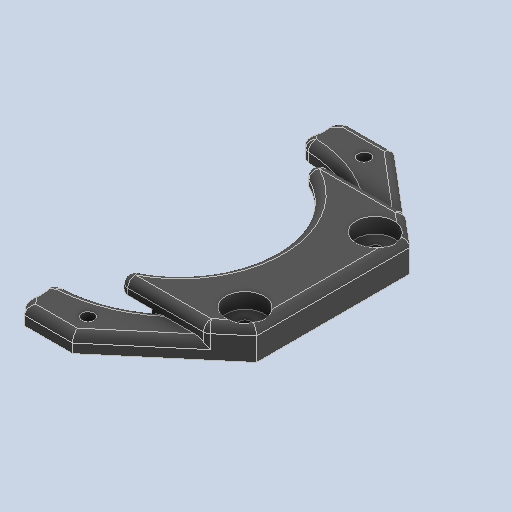
# Autodesk Inventor part: joit_cover_arm_upper
Saved by Autodesk Inventor 2026.1 (Build 301233020, 233B)
## iProperties
Created: 2024-02-14
Part Number: joit_cover_arm_upper
Material: 一般
Document SubType Name: Modeling
Designer: hibik
Density: 1 g/cm^3
Appearance: 既定
Author: hibik
Autodesk Inventor part; units mm, degrees
ref_plane "YZ Plane" through (0, 0, 0) normal (1, 0, 0) x (0, 1, 0)
ref_plane "XZ Plane" through (0, 0, 0) normal (0, 1, 0) x (-1, 0, 0)
ref_plane "XY Plane" through (0, 0, 0) normal (0, 0, 1) x (1, 0, 0)
sketch "スケッチ1" plane through (0, 0, 0) normal (0, 1, 0) x (-1, 0, 0)
  line L0 (24, 0) -> (0, 0)
  line L1 (0, 0) -> (0, -26)
  line L2 (0, -26) -> (24, -26)
  line L3 (24, -26) -> (24, 0)
  circle A0 centre (24, -13) radius 13 construction
  circle A1 centre (24, -13) radius 12.5
  circle A2 centre (24, -13) radius 16
  point P0 (24, -25.5)
  point P1 (24, -0.5)
  point P2 (14.672621, 0)
  point P3 (14.672621, -26)
  dimension "d0" = 26
  dimension "d1" = 24
  dimension "d2" = 25
  dimension "d3" = 32
  constraints: 8 end point, 3 centre point, 3 coincident, 2 parallel, 1 horizontal, 1 midpoint, 1 perpendicular, 1 tangent
  measures "d0" distance of L2.end L0.start
  measures "d1" distance of L1.end L2.end
  measures "d2" diameter of A1
  measures "d3" diameter of A2
extrude "押し出し1" add sketch "スケッチ1" along normal blind 4 contours L3 A1 L2 A2 L0 | A2 L2 L1 L0 picked at (14.087861, -23.933914)
extrude "押し出し2" cut sketch "スケッチ1" along normal blind 2.2 contours L3 A1 L2 A2 L0 picked at (14.087861, -23.933914)
fillet "フィレット1" radius 1 4 edges at (-24, 3.1, -0.5) (-24, 3.1, 0) (-24, 3.1, -26) (-24, 3.1, -25.5)
sketch "スケッチ8" plane through (0, 0, 0) normal (0, -1, 0) x (1, 0, 0)
  line L0 (-4, -3) -> (-4, -5.236068)
  line L1 (-5.661079, -1.594472) -> (-4, -3)
  line L2 (-4, -20.763932) -> (-4, -23)
  line L3 (-4, -23) -> (-5.661079, -24.405528)
  line L4 (-15.355616, -32.608598) -> (-17, -34)
  line L5 (-17, 8) -> (-15.355616, 6.608598)
  line L6 (-17, -34) -> (-45, -34)
  line L7 (-45, 8) -> (-17, 8)
  line L8 (-5.661079, -1.594472) -> (-15.355616, 6.608598)
  line L9 (-4, -5.236068) -> (-4, -20.763932)
  line L10 (-5.661079, -24.405528) -> (-15.355616, -32.608598)
  arc A0 (-18.273464, -24.111111) -> (-18.273464, -1.888889) centre (-24, -13) ccw
  circle A1 centre (-24, -13) radius 12.5
  line L11 (-23.274102, -34) -> (-25.857871, -30.946455)
  line L12 (-25.857871, -30.946455) -> (-15.925722, -22.542329)
  line L13 (-23.274102, 8) -> (-25.857871, 4.946455)
  line L14 (-25.857871, 4.946455) -> (-15.925722, -3.457671)
  arc A2 (-14.672621, -26) -> (-14.672621, 0) centre (-24, -13) ccw
  line L15 (0, -26) -> (-14.672621, -26)
  line L16 (0, 0) -> (0, -26)
  line L17 (-14.672621, 0) -> (0, 0)
  line L18 (-14.672621, -26) -> (-17.815342, -26)
  line L19 (-14.672621, -26) -> (-20.012061, -26)
  line L20 (-14.672621, 0) -> (-20.012061, 0)
  circle A3 centre (-24, -13) radius 16
  point P0 (-7.545455, -26)
  point P1 (-7.545455, 0)
  point P2 (-23.550037, 2.993672)
  point P3 (-14.672621, 0)
  point P4 (-23.550037, -28.993672)
  dimension "d35" = 4
  constraints: 18 end point, 4 point on line, 3 parallel, 2 centre point, 2 coincident, 2 collinear, 2 concentric, 2 perpendicular, 2 point on circle, 2 tangent, 1 vertical, 1 vertical alignment
  measures "d35" distance from line of L13.start L14
extrude "押し出し10" add sketch "スケッチ8" against normal up to surface (2.2 mm away) contours L17 A3 L14 L13 L7 L5 L8 | L10 L4 L6 L11 L12 A3 L15
sketch "スケッチ9" plane through (0, 0, 0) normal (0, -1, 0) x (1, 0, 0)
  line L0 (-4, -3) -> (-4, -5.236068)
  line L1 (-5.661079, -1.594472) -> (-4, -3)
  line L2 (-4, -20.763932) -> (-4, -23)
  line L3 (-4, -23) -> (-5.661079, -24.405528)
  line L4 (-17.815342, 0) -> (0, 0)
  line L5 (-7.545455, 0) -> (-5.661079, -1.594472)
  line L6 (-4, -5.236068) -> (-4, -20.763932)
  line L7 (-5.661079, -24.405528) -> (-7.545455, -26)
  line L8 (0, -26) -> (-7.545455, -26)
  line L9 (0, 0) -> (0, -26)
  line L10 (-7.545455, 0) -> (0, 0)
  line L11 (-7.545455, 0) -> (-17, 8)
  line L12 (-17, 8) -> (-23.274102, 8)
  line L13 (-23.274102, 8) -> (-25.857871, 4.946455)
  line L14 (-25.857871, 4.946455) -> (-23.550037, 2.993672)
  line L15 (-23.550037, -28.993672) -> (-25.857871, -30.946455)
  line L16 (-25.857871, -30.946455) -> (-23.274102, -34)
  line L17 (-23.274102, -34) -> (-17, -34)
  line L18 (-17, -34) -> (-7.545455, -26)
  arc A0 (-23.550037, -28.993672) -> (-23.550037, 2.993672) centre (-24, -13) ccw
  constraints: 6 end point, 1 coincident, 1 collinear, 1 perpendicular, 1 point on line
extrude "押し出し11" cut sketch "スケッチ9" against normal through all contours L1 L5 L4 L9 L8 L7 L3 L2 L6 L0
fillet "フィレット5" radius 1 22 edges at (-12.2727, 2.2, -30) (-20.1371, 2.2, -34) (-24.566, 2.2, -32.4732) (-24.704, 2.2, -29.9701) (-5.7727, 4, -24.5) (-4, 4, -13) (-5.7727, 4, -1.5) (-12.2727, 2.2, 4) (-20.1371, 2.2, 8) (-24.566, 2.2, 6.4732) (-24.704, 2.2, 3.9701) (-18.7872, 4, -0.7643) (-11.5, 4, -13) (-18.7872, 4, -25.2357) (-12.6804, 4, -26) (-12.6804, 4, 0) (-7.5455, 3.1, 0) (-7.5455, 3.1, -26) (-23.55, 1.1, 2.9937) (-23.55, 1.1, -28.9937) (-18.8873, 2.2, -28.1611) (-18.8873, 2.2, 2.1611)
sketch "スケッチ10" plane through (0, 0, 0) normal (0, -1, 0) x (1, 0, 0)
  circle A0 centre (-7.005883, -4.502942) radius 0.8
  circle A1 centre (-7.005883, -21.497058) radius 0.8
  circle A2 centre (-17.991672, -31.024983) radius 0.8
  circle A3 centre (-17.991672, 5.024983) radius 0.8
  point P0 (0, 0)
extrude "押し出し12" cut sketch "スケッチ10" against normal through all
sketch "スケッチ11" plane through (0, 4, 0) normal (0, 1, 0) x (1, 0, 0)
  circle A0 centre (-7.005883, 4.502942) radius 0.8
  circle A1 centre (-7.005883, 21.497058) radius 0.8
  circle A2 centre (-7.005883, 4.502942) radius 2.5
  circle A3 centre (-7.005883, 21.497058) radius 2.5
  point P0 (0, 0)
  dimension "d43" = 5
  dimension "d44" = 5
  constraints: 2 centre point, 2 coincident
  measures "d43" diameter of A2
  measures "d44" diameter of A3
extrude "押し出し13" cut sketch "スケッチ11" against normal blind 2
sketch "スケッチ12" plane through (0, 0, 0) normal (0, -1, 0) x (1, 0, 0)
  circle A0 centre (-27, -31.5) radius 1 projected
  circle A1 centre (-27, 5.5) radius 1 projected
  circle A2 centre (-27, 5.5) radius 3.5
  circle A3 centre (-27, -31.5) radius 3.5
  point P0 (0, 0)
  dimension "d47" = 7
  dimension "d48" = 7
  constraints: 2 centre point, 2 coincident
  measures "d47" diameter of A2
  measures "d48" diameter of A3
extrude "押し出し14" cut sketch "スケッチ12" against normal through all contours A0 | A1 | A2 | A3
